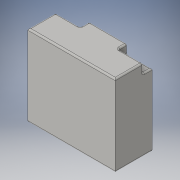
# Autodesk Inventor part: FRC Battery
Saved by Autodesk Inventor 2016 (Build 200138000, 138)
## iProperties
Created: 2018-07-06
Part Number: FRC Battery
Material: Generic
Document SubType Name: Modeling
Designer: Kade
Density: 1 g/cm^3
Appearance: Default
Author: Kade
Autodesk Inventor part; units mm, degrees
ref_plane "YZ Plane" through (0, 0, 0) normal (1, 0, 0) x (0, 1, 0)
ref_plane "XZ Plane" through (0, 0, 0) normal (0, 1, 0) x (-1, 0, 0)
ref_plane "XY Plane" through (0, 0, 0) normal (0, 0, 1) x (1, 0, 0)
sketch "Sketch1" plane through (0, 0, 0) normal (0, 1, 0) x (-1, 0, 0)
  line L0 (0, 0) -> (180.34, 0)
  line L1 (180.34, 0) -> (180.34, -76.2)
  line L2 (180.34, -76.2) -> (0, -76.2)
  line L3 (0, -76.2) -> (0, 0)
  dimension "d0" = 180.34
  dimension "d1" = 76.2
  constraints: 8 end point, 2 parallel, 1 horizontal, 1 perpendicular
  measures "d0" distance of L1.end L2.end
  measures "d1" distance of L0.end L1.end
extrude "Extrusion1" add sketch "Sketch1" along normal blind 167.64
fillet "Fillet1" radius 3.175 8 edges at (-90.17, 167.64, 0) (-180.34, 167.64, -38.1) (-90.17, 167.64, -76.2) (0, 167.64, -38.1) (-90.17, 0, -76.2) (-180.34, 0, -38.1) (-90.17, 0, 0) (0, 0, -38.1)
sketch "Sketch2" plane through (0, 3.175, -76.2) normal (1, 0, 0) x (0, 0, -1)
  line L0 (0, 164.465) -> (-19.05, 164.465)
  line L1 (-19.05, 164.465) -> (-19.05, 145.415)
  line L2 (-19.05, 145.415) -> (0, 145.415)
  line L3 (0, 145.415) -> (0, 164.465)
  line L4 (0, 164.465) -> (-19.05, 164.465)
  line L5 (-19.05, 164.465) -> (-19.05, 145.415)
  line L6 (-19.05, 145.415) -> (0, 145.415)
  line L7 (0, 145.415) -> (0, 164.465)
  point P0 (-76.2, -3.175)
  dimension "d5" = 19.05
  dimension "d6" = 19.05
  constraints: 16 end point, 4 parallel, 2 horizontal, 2 perpendicular
  measures "d5" distance of L2.end L1.end
  measures "d6" distance of L1.end L0.end
extrude "Extrusion2" cut sketch "Sketch2" against normal blind 50.8
sketch "Sketch3" plane through (-180.34, 3.175, 0) normal (-1, 0, 0) x (0, 0, 1)
  line L0 (-76.2, 164.465) -> (-57.15, 164.465)
  line L1 (-57.15, 164.465) -> (-57.15, 145.415)
  line L2 (-57.15, 145.415) -> (-76.2, 145.415)
  line L3 (-76.2, 145.415) -> (-76.2, 164.465)
  point P0 (0, -3.175)
  dimension "d9" = 19.05
  dimension "d10" = 19.05
  constraints: 8 end point, 2 parallel, 1 horizontal, 1 perpendicular
  measures "d9" distance of L1.end L2.end
  measures "d10" distance of L0.end L1.end
extrude "Extrusion3" cut sketch "Sketch3" against normal blind 50.8
fillet "Fillet2" radius 3.175 22 edges at (-154.94, 148.59, -57.15) (-129.54, 148.59, -66.675) (-129.54, 158.115, -57.15) (-179.4101, 166.7101, -57.15) (-180.34, 156.5275, -57.15) (-153.3525, 167.64, -57.15) (-129.54, 166.7101, -75.2701) (-129.54, 156.5275, -76.2) (-129.54, 167.64, -65.0875) (-154.94, 148.59, -76.2) (-180.34, 148.59, -66.675) (-25.4, 148.59, -76.2) (-50.8, 166.7101, -75.2701) (-50.8, 167.64, -65.0875) (-50.8, 156.5275, -76.2) (-0.9299, 166.7101, -57.15) (0, 156.5275, -57.15) (-26.9875, 167.64, -57.15) (0, 148.59, -66.675) (-25.4, 148.59, -57.15) (-50.8, 148.59, -66.675) (-50.8, 158.115, -57.15)
body "Solid1"
